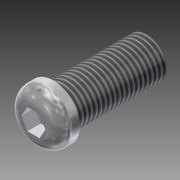
# Autodesk Inventor part: M3x13
Saved by Autodesk Inventor 2015 (Build 190159000, 159)
## iProperties
Created: 2017-01-16
Part Number: M3x13
Material: Generic
Document SubType Name: Modeling
Designer: Per
Density: 1 g/cm^3
Appearance: Aluminum - Dark
Author: Per
Autodesk Inventor part; units mm, degrees
ref_plane "YZ Plane" through (0, 0, 0) normal (1, 0, 0) x (0, 1, 0)
ref_plane "XZ Plane" through (0, 0, 0) normal (0, 1, 0) x (-1, 0, 0)
ref_plane "XY Plane" through (0, 0, 0) normal (0, 0, 1) x (1, 0, 0)
sketch "Sketch1" plane through (0, 0, 0) normal (0, 1, 0) x (-1, 0, 0)
  circle A0 centre (0, 0) radius 2
  dimension "d0" = 4
  constraints: 1 centre point, 1 coincident
  measures "d0" diameter of A0
extrude "Extrusion1" add sketch "Sketch1" along normal blind 1.5
sketch "Sketch2" plane through (0, 1.5, 0) normal (0, 1, 0) x (1, 0, 0)
  circle A0 centre (0, 0) radius 1.5
  dimension "d3" = 3
  constraints: 1 centre point, 1 coincident
  measures "d3" diameter of A0
extrude "Extrusion2" add sketch "Sketch2" along normal blind 7
sketch "Sketch3" plane through (0, 0, 0) normal (0, -1, 0) x (1, 0, 0)
  line L0 (0.905, 0) -> (0.4525, -0.7838)
  line L1 (0.4525, -0.7838) -> (-0.4525, -0.7838)
  line L2 (-0.4525, -0.7838) -> (-0.905, 0)
  line L3 (-0.905, 0) -> (-0.4525, 0.7838)
  line L4 (-0.4525, 0.7838) -> (0.4525, 0.7838)
  line L5 (0.4525, 0.7838) -> (0.905, 0)
  point P0 (0, 0)
  point P1 (0, 0)
  constraints: 12 end point, 1 coincident, 13 other
extrude "Extrusion3" cut sketch "Sketch3" against normal blind 1
fillet "Fillet1" radius 1 1 edges at (2, 0, 0)
thread "Thread1" size "M3x0.35" class "6g" standard "ANSI Metric M Profile" full length
body "Solid1"
